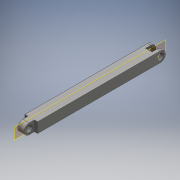
# Autodesk Inventor part: ServoLinkage
Saved by Autodesk Inventor 2016 (Build 200138000, 138)
## iProperties
Created: 2016-11-02
Part Number: ServoLinkage
Material: Generic
Document SubType Name: Modeling
Designer: mattc
Density: 1 g/cm^3
Appearance: Smooth - Medium Gray
Author: mattc
Autodesk Inventor part; units mm, degrees
ref_plane "YZ Plane" through (0, 0, 0) normal (1, 0, 0) x (0, 1, 0)
ref_plane "XZ Plane" through (0, 0, 0) normal (0, 1, 0) x (-1, 0, 0)
ref_plane "XY Plane" through (0, 0, 0) normal (0, 0, 1) x (1, 0, 0)
sketch "Sketch1" plane through (0, 0, 0) normal (1, 0, 0) x (0, 1, 0)
  circle A0 centre (0, 0) radius 2.5
  arc A1 (0, 4) -> (0, -4) centre (0, 0) ccw
  line L0 (0, 4) -> (100, 4)
  line L1 (100, -4) -> (0, -4)
  arc A2 (100, -4) -> (100, 4) centre (100, 0) ccw
  circle A3 centre (100, 0) radius 2.5
  dimension "d0" = 5
  dimension "d1" = 8
  dimension "d3" = 100
  dimension "d4" = 8
  dimension "d5" = 5
  constraints: 4 centre point, 4 end point, 4 point on circle, 3 coincident, 3 tangent, 1 horizontal, 1 parallel
  measures "d0" diameter of A0
  measures "d1" diameter of A1
  measures "d3" distance of L0.start L0.end
  measures "d4" distance of L0.end L1.start
  measures "d5" diameter of A3
extrude "Extrusion1" add sketch "Sketch1" along normal blind 10
ref_plane "Work Plane1" through (5, 0, 0) normal (1, 0, 0) x (0, 0, -1)
sketch "Sketch2" plane through (5, 0, 0) normal (1, 0, 0) x (0, 0, -1)
  circle A0 centre (0, 100) radius 2.5 projected
  arc A1 (4, 100) -> (-4, 100) centre (0, 100) ccw projected
  line L0 (0, 104) -> (5, 104)
  line L1 (5, 104) -> (-5, 104)
  line L2 (-5, 104) -> (-5, 96)
  line L3 (-5, 96) -> (5, 96)
  line L4 (5, 96) -> (5, 104)
  point P0 (0, 0)
  dimension "d9" = 5
  dimension "d10" = 10
  dimension "d11" = 8
  constraints: 10 end point, 2 horizontal, 2 parallel, 1 perpendicular, 1 point on circle, 1 tangent
  measures "d9" distance of L0.start L0.end
  measures "d10" distance of L3.end L2.end
  measures "d11" distance of L2.end L1.end
extrude "Extrusion2" cut sketch "Sketch2" along normal mid plane 5
sketch "Sketch4" plane through (10, 0, 0) normal (1, 0, 0) x (0, 0, -1)
  line L0 (5, -4) -> (-5, -4)
  line L1 (-5, -4) -> (-5, 4)
  line L2 (-5, 4) -> (5, 4)
  line L3 (5, 4) -> (5, -4)
  point P0 (0, 0)
  dimension "d19" = 10
  dimension "d20" = 8
  constraints: 8 end point, 2 parallel, 1 horizontal, 1 perpendicular
  measures "d19" distance of L1.end L2.end
  measures "d20" distance of L0.end L1.end
extrude "Extrusion4" cut sketch "Sketch4" against normal blind 2.5
sketch "Sketch5" plane through (0, 0, 0) normal (-1, 0, 0) x (0, 0, 1)
  line L0 (5, -4) -> (-5, -4)
  line L1 (-5, -4) -> (-5, 4)
  line L2 (-5, 4) -> (5, 4)
  line L3 (5, 4) -> (5, -4)
  point P0 (0, 0)
  dimension "d23" = 10
  dimension "d24" = 8
  constraints: 8 end point, 2 parallel, 1 horizontal, 1 perpendicular
  measures "d23" distance of L1.end L2.end
  measures "d24" distance of L0.end L1.end
extrude "Extrusion5" cut sketch "Sketch5" against normal blind 2.5
equation "\"d5\" = d0"
body "Solid1"
